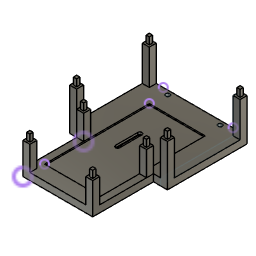
WRO BOTTOM LAYER_ (Autodesk Fusion 360 design; units mm, degrees)
Autodesk Fusion 360 part; units mm, degrees
note: some values were not read from the file. Set by a fixed rule: which sketch regions a step uses.
sketch "Sketch1" plane through (0, 0, 0) normal (1, 0, 0) x (0, 1, 0)
  line L0 (0, 0) -> (-25, 0)
  line L1 (-25, 0) -> (29, 0)
  line L2 (29, 0) -> (32, 0)
  line L3 (32, 0) -> (32, 30)
  line L4 (32, 30) -> (67, 30)
  line L5 (67, 30) -> (67, 35)
  line L6 (67, 35) -> (27, 35)
  line L7 (27, 35) -> (27, 5)
  line L8 (27, 5) -> (-25, 5)
  line L9 (-25, 5) -> (-25, 0)
  dimension "d1" = 25
  dimension "d2" = 54
  dimension "d3" = 3
  dimension "d4" = 30
  dimension "d5" = 35
  dimension "d6" = 5
  dimension "d7" = 40
  dimension "d8" = 30
  dimension "d9" = 52
  constraint coincident L0.start origin
  constraint horizontal L0
  constraint parallel L0 L1
  constraint parallel L1 L2
  constraint perpendicular L2 L3
  constraint perpendicular L3 L4
  constraint perpendicular L4 L5
  constraint perpendicular L5 L6
  constraint perpendicular L1 L7
  constraint perpendicular L7 L8
  measures "d1" distance of L0.start L0.end
  measures "d2" distance of L0.end L1.end
  measures "d3" distance of L1.end L2.end
  measures "d4" distance of L2.end L3.end
  measures "d5" distance of L3.end L4.end
  measures "d6" distance of L4.end L5.end
  measures "d7" distance of L5.end L6.end
  measures "d8" distance of L6.end L7.end
  measures "d9" distance of L7.end L8.end
extrude "Extrude1" add sketch "Sketch1" along normal blind 30 and the other way blind 30 makes body 1
sketch "Sketch2" plane through (0, 27, 0) normal (0, -1, 0) x (1, 0, 0)
  line L0 (-30, 5) -> (30, 5)
  line L1 (30, 5) -> (30, 35)
  line L2 (30, 35) -> (-30, 35)
  line L3 (-30, 35) -> (-30, 5)
  line L4 (-25, 5) -> (25, 5)
  line L5 (25, 5) -> (25, 30)
  line L6 (25, 30) -> (-25, 30)
  line L7 (-25, 30) -> (-25, 5)
  constraint horizontal L4
  constraint vertical L5
  constraint horizontal L6
  constraint vertical L7
  constraint coincident L0 L4.start
extrude "Extrude2" cut sketch "Sketch2" against normal blind 430 contours L0 L4 L5 L6 L7 bodies 1
sketch "Sketch3" plane through (0, 0, 5) normal (0, 0, 1) x (-1, 0, 0)
  line L0 (30, 25) -> (-30, 25)
  line L1 (-30, 25) -> (-30, -27)
  line L2 (-30, -27) -> (-25, -27)
  line L3 (-25, -27) -> (-25, -32)
  line L4 (-25, -32) -> (25, -32)
  line L5 (25, -32) -> (25, -27)
  line L6 (25, -27) -> (30, -27)
  line L7 (30, -27) -> (30, 25)
  line L8 (30, 0) -> (20, 0)
  line L9 (20, 0) -> (20, -20)
  line L10 (20, -20) -> (-20, -20)
  line L11 (-20, -20) -> (-20, 55)
  line L12 (-20, 55) -> (20, 55)
  line L13 (20, 55) -> (20, -20)
  dimension "d16" = 10
  dimension "d17" = 40
  dimension "d18" = 75
  constraint coincident L7 L8.start
  constraint perpendicular L7 L8
  constraint perpendicular L8 L9
  constraint horizontal L10
  constraint vertical L11
  constraint horizontal L12
  constraint vertical L13
  measures "d16" distance of L8.start L8.end
  measures "d17" distance of L9.end L10.end
  measures "d18" distance of L9.end L12.end
sketch "Sketch4" plane through (0, -25, 0) normal (0, -1, 0) x (1, 0, 0)
  line L0 (-30, 0) -> (30, 0)
  line L1 (30, 0) -> (30, 5)
  line L2 (30, 5) -> (-30, 5)
  line L3 (-30, 5) -> (-30, 0)
  line L4 (-30, 0) -> (-25, 0)
  line L5 (-25, 0) -> (25, 0)
  line L6 (25, 0) -> (25, 5)
  line L7 (25, 5) -> (-25, 5)
  line L8 (-25, 5) -> (-25, 0)
  dimension "d19" = 5
  dimension "d20" = 50
  dimension "d21" = 5
  constraint coincident L0.start L3.end
  constraint perpendicular L3 L4
  constraint horizontal L5
  constraint vertical L6
  constraint horizontal L7
  constraint vertical L8
  measures "d19" distance of L0.start L4.end
  measures "d20" distance of L4.end L5.end
  measures "d21" distance of L4.end L7.end
extrude "Extrude3" add sketch "Sketch4" along normal blind 43.5 contours L0 L2 L5 L6 L7 L8 bodies 1
extrude "Extrude4" cut sketch "Sketch3" against normal blind 1 contours L0 L9 L10 L11 L13 | L0 L11 L12 L13 bodies 1
sketch "Sketch5" plane through (30, 0, 0) normal (1, 0, 0) x (0, 1, 0)
  line L0 (-25, 5) -> (-25, 0)
  line L1 (-25, 0) -> (32, 0)
  line L2 (32, 0) -> (32, 30)
  line L3 (32, 30) -> (67, 30)
  line L4 (67, 30) -> (67, 35)
  line L5 (67, 35) -> (27, 35)
  line L6 (27, 35) -> (27, 5)
  line L7 (27, 5) -> (-25, 5)
  line L8 (67, 30) -> (62, 30)
  line L9 (62, 30) -> (62, 5)
  line L10 (62, 5) -> (67, 5)
  line L11 (67, 5) -> (67, 30)
  line L12 (62, 5) -> (78, 5)
  line L13 (78, 5) -> (78, 10)
  line L14 (78, 10) -> (62, 10)
  line L15 (62, 10) -> (62, 5)
  dimension "d26" = 5
  dimension "d27" = 25
  dimension "d28" = 16
  dimension "d29" = 5
  constraint horizontal L8
  constraint vertical L9
  constraint horizontal L10
  constraint vertical L11
  constraint coincident L3.end L4.start
  constraint horizontal L12
  constraint vertical L13
  constraint horizontal L14
  constraint vertical L15
  measures "d26" distance of L3.end L8.end
  measures "d27" distance of L3.end L10.end
  measures "d28" distance of L9.end L12.end
  measures "d29" distance of L9.end L14.end
extrude "Extrude5" add sketch "Sketch5" against normal blind 60 contours L3 L8 L9 L11 L14 | L9 L10 L11 L12 L14 L15 | L11 L12 L13 L14 bodies 1
sketch "Sketch6" plane through (30, 0, 0) normal (1, 0, 0) x (0, 1, 0)
  line L0 (-25, 5) -> (-25, 0)
  line L1 (-25, 0) -> (32, 0)
  line L2 (32, 0) -> (32, 30)
  line L3 (32, 30) -> (62, 30)
  line L4 (62, 30) -> (62, 5)
  line L5 (62, 5) -> (78, 5)
  line L6 (78, 5) -> (78, 10)
  line L7 (78, 10) -> (67, 10)
  line L8 (67, 10) -> (67, 35)
  line L9 (67, 35) -> (27, 35)
  line L10 (27, 35) -> (27, 5)
  line L11 (27, 5) -> (-25, 5)
  line L12 (62, 30) -> (99.4682, 30)
  line L13 (99.4682, 30) -> (99.4682, 1.0455)
  line L14 (99.4682, 1.0455) -> (62, 1.0455)
  line L15 (62, 1.0455) -> (62, 30)
  constraint horizontal L12
  constraint vertical L13
  constraint horizontal L14
  constraint vertical L15
  constraint coincident L3.end L4.start
extrude "Extrude6" cut sketch "Sketch6" against normal blind 5 contours L4 L5 L6 L7 L8 L12 L15 bodies 1
sketch "Sketch7" plane through (-30, 0, 0) normal (-1, 0, 0) x (0, -1, 0)
  line L0 (25, 0) -> (25, 5)
  line L1 (25, 5) -> (-27, 5)
  line L2 (-27, 5) -> (-27, 35)
  line L3 (-27, 35) -> (-67, 35)
  line L4 (-67, 35) -> (-67, 10)
  line L5 (-67, 10) -> (-78, 10)
  line L6 (-78, 10) -> (-78, 5)
  line L7 (-78, 5) -> (-62, 5)
  line L8 (-62, 5) -> (-62, 30)
  line L9 (-62, 30) -> (-32, 30)
  line L10 (-32, 30) -> (-32, 0)
  line L11 (-32, 0) -> (25, 0)
  line L12 (-62, 30) -> (-89.4119, 30)
  line L13 (-89.4119, 30) -> (-89.4119, -1.5433)
  line L14 (-89.4119, -1.5433) -> (-62, -1.5433)
  line L15 (-62, -1.5433) -> (-62, 30)
  constraint horizontal L12
  constraint vertical L13
  constraint horizontal L14
  constraint vertical L15
  constraint coincident L8.end L9.start
extrude "Extrude7" cut sketch "Sketch7" against normal blind 5 contours L4 L5 L6 L7 L8 L12 L15 bodies 1
sketch "Sketch8" plane through (0, 67, 0) normal (0, 1, 0) x (-1, 0, 0)
  line L0 (25, 30) -> (30, 30)
  line L1 (30, 30) -> (30, 35)
  line L2 (30, 35) -> (-30, 35)
  line L3 (-30, 35) -> (-30, 30)
  line L4 (-30, 30) -> (-25, 30)
  line L5 (-25, 30) -> (-25, 10)
  line L6 (-25, 10) -> (25, 10)
  line L7 (25, 10) -> (25, 30)
  line L8 (-25, 10) -> (-20, 10)
  line L9 (-20, 10) -> (20, 10)
  line L10 (20, 10) -> (20, 30)
  line L11 (20, 30) -> (-20, 30)
  line L12 (-20, 30) -> (-20, 10)
  dimension "d36" = 5
  dimension "d37" = 40
  constraint coincident L5.end L6.start
  constraint perpendicular L5 L8
  constraint horizontal L9
  constraint vertical L10
  constraint horizontal L11
  constraint vertical L12
  measures "d36" distance of L5.end L8.end
  measures "d37" distance of L8.end L9.end
extrude "Extrude8" cut sketch "Sketch8" against normal blind 16 contours L6 L9 L10 L11 L12 bodies 1
sketch "Sketch9" plane through (0, 0, 10) normal (0, 0, 1) x (-1, 0, 0)
  line L0 (25, -78) -> (25, -67)
  line L1 (25, -67) -> (20, -67)
  line L2 (20, -67) -> (20, -62)
  line L3 (20, -62) -> (-20, -62)
  line L4 (-20, -62) -> (-20, -67)
  line L5 (-20, -67) -> (-25, -67)
  line L6 (-25, -67) -> (-25, -78)
  line L7 (-25, -78) -> (25, -78)
  line L8 (-14, -62) -> (-14, -69.25)
  line L9 (-14, -69.25) -> (-14, -70)
  line L10 (-25, -70.7379) -> (0, -70.7379)
  line L11 (0, -70.7379) -> (-7.25, -70.7379)
  line L12 (-14, -70) -> (-7.25, -70)
  line L13 (-7.25, -70) -> (-7.25, -70.7379)
  circle A0 centre (-7.25, -70) radius 0.75
  line L14 (-7.25, -70) -> (7.25, -70)
  circle A1 centre (7.25, -70) radius 0.75
  dimension "d40" = 7.25
  dimension "d41" = 0.75
  dimension "d42" = 25
  dimension "d43" = 7.25
  dimension "d44" = 1.5
  dimension "d45" = 14.5
  dimension "d46" = 1.5
  constraint vertical L8
  constraint coincident L3 L8.start
  constraint perpendicular L7 L9
  constraint coincident L6 L10.start
  constraint perpendicular L0 L10
  constraint parallel L10 L11
  constraint perpendicular L9 L12
  constraint perpendicular L11 L13
  constraint coincident L12.end L13.start
  constraint perpendicular L13 L14
  constraint coincident L14.end A1.centre
  measures "d40" distance of L8.start L8.end
  measures "d41" distance of L8.end L9.end
  measures "d42" distance of L10.start L10.end
  measures "d43" distance of L10.end L11.end
  measures "d44" diameter of A0
  measures "d45" distance of L12.end L14.end
  measures "d46" diameter of A1
extrude "Extrude9" cut sketch "Sketch9" against normal blind 1000000 contours L10 L12 L13 A0 | L10 L11 L13 A0 L14 | L12 A0 L14 | A1 bodies 1
sketch "Sketch10" plane through (0, 0, 5) normal (0, 0, 1) x (-1, 0, 0)
  line L0 (-20, -20) -> (-20, 55)
  line L1 (-20, 55) -> (20, 55)
  line L2 (20, 55) -> (20, -20)
  line L3 (20, -20) -> (-20, -20)
  line L4 (-25, 25) -> (-30, 25)
  line L5 (-30, 25) -> (-30, -27)
  line L6 (-30, -27) -> (-25, -27)
  line L7 (-25, -27) -> (-25, -32)
  line L8 (-25, -32) -> (25, -32)
  line L9 (25, -32) -> (25, -27)
  line L10 (25, -27) -> (30, -27)
  line L11 (30, -27) -> (30, 25)
  line L12 (30, 25) -> (25, 25)
  line L13 (25, 25) -> (25, 68.5)
  line L14 (25, 68.5) -> (-25, 68.5)
  line L15 (-25, 68.5) -> (-25, 25)
  line L16 (15.6178, -32) -> (15.6178, -29)
  line L17 (15.6178, -29) -> (-84.3822, -29)
  line L18 (15.6178, -29) -> (37, -29)
  line L19 (25, -29) -> (0, -29)
  line L20 (0, -29) -> (18.75, -29)
  line L21 (18.75, -29) -> (-18.75, -29)
  circle A0 centre (18.75, -29) radius 1
  circle A1 centre (-18.75, -29) radius 1
  dimension "d49" = 3
  dimension "d50" = 100
  dimension "d51" = 25
  dimension "d52" = 18.75
  dimension "d53" = 37.5
  dimension "d54" = 2
  dimension "d55" = 2
  constraint coincident L8 L16.start
  constraint perpendicular L8 L16
  constraint perpendicular L16 L17
  constraint perpendicular L16 L18
  constraint coincident L18 L19.start
  constraint coincident L9 L19.start
  constraint perpendicular L7 L19
  constraint horizontal L20
  constraint perpendicular L16 L21
  constraint coincident L20.end L21.start
  constraint coincident L21.end A1.centre
  measures "d49" distance of L16.start L16.end
  measures "d50" distance of L16.end L17.end
  measures "d51" distance of L19.start L19.end
  measures "d52" distance of L19.end L20.end
  measures "d53" distance of L20.end L21.end
  measures "d54" diameter of A0
  measures "d55" diameter of A1
extrude "Extrude10" cut sketch "Sketch10" against normal blind 1000 contours L17 L21 A1 | L17 L21 A1 | L18 L19 L20 L21 A0 | L18 L19 L20 L21 A0 bodies 1
sketch "Sketch11" plane through (0, 0, 5) normal (0, 0, 1) x (-1, 0, 0)
  circle A0 centre (-18.75, -29) radius 1
  circle A1 centre (18.75, -29) radius 1
  line L0 (-20, -20) -> (-20, 55)
  line L1 (-20, 55) -> (20, 55)
  line L2 (20, 55) -> (20, -20)
  line L3 (20, -20) -> (-20, -20)
  line L4 (-25, 25) -> (-30, 25)
  line L5 (-30, 25) -> (-30, -27)
  line L6 (-30, -27) -> (-25, -27)
  line L7 (-25, -27) -> (-25, -32)
  line L8 (-25, -32) -> (25, -32)
  line L9 (25, -32) -> (25, -27)
  line L10 (25, -27) -> (30, -27)
  line L11 (30, -27) -> (30, 25)
  line L12 (30, 25) -> (25, 25)
  line L13 (25, 25) -> (25, 68.5)
  line L14 (25, 68.5) -> (-25, 68.5)
  line L15 (-25, 68.5) -> (-25, 25)
  circle A2 centre (18.75, -29) radius 1.5
  circle A3 centre (-18.75, -29) radius 1.5
  dimension "d58" = 3
  dimension "d59" = 3
  constraint concentric A1 A2
  constraint concentric A0 A3
  measures "d58" diameter of A2
  measures "d59" diameter of A3
extrude "Extrude11" cut sketch "Sketch11" against normal blind 2.5 contours A2 | A3 bodies 1
extrude "Extrude12" add 1 faces at (-6.6667, -5, 4) along direction (0, 0, 1) blind 1 on bodies 1 bodies 1
sketch "Sketch12" plane through (0, 0, 5) normal (0, 0, 1) x (-1, 0, 0)
  circle A0 centre (18.75, -29) radius 1.5
  circle A1 centre (-18.75, -29) radius 1.5
  line L0 (-25, 25) -> (-30, 25)
  line L1 (-30, 25) -> (-30, -27)
  line L2 (-30, -27) -> (-25, -27)
  line L3 (-25, -27) -> (-25, -32)
  line L4 (-25, -32) -> (25, -32)
  line L5 (25, -32) -> (25, -27)
  line L6 (25, -27) -> (30, -27)
  line L7 (30, -27) -> (30, 25)
  line L8 (30, 25) -> (25, 25)
  line L9 (25, 25) -> (25, 68.5)
  line L10 (25, 68.5) -> (-25, 68.5)
  line L11 (-25, 68.5) -> (-25, 25)
  line L12 (18.75, -29) -> (17.25, -29)
  line L13 (17.25, -29) -> (5.725, -29)
  line L14 (5.725, -29) -> (5.725, 21)
  circle A2 centre (5.7328, 20) radius 1
  circle A3 centre (5.7328, 20) radius 1
  line L15 (5.7328, 20) -> (4.7328, 20)
  line L16 (4.7328, 20) -> (6.7328, 20)
  line L17 (6.7328, 20) -> (6.7328, 4)
  line L18 (6.7328, 4) -> (4.7328, 4)
  line L19 (4.7328, 4) -> (4.7328, 20)
  circle A4 centre (5.7328, 4) radius 1
  dimension "d64" = 11.525
  dimension "d65" = 50
  dimension "d66" = 2
  dimension "d67" = 2
  dimension "d68" = 16
  dimension "d69" = 2
  constraint coincident A0.centre L12.start
  constraint coincident A0 L12.end
  constraint horizontal L12
  constraint parallel L12 L13
  constraint perpendicular L13 L14
  constraint coincident L14.end A2
  constraint concentric A2 A3
  constraint coincident A2.centre A3.centre
  constraint coincident A3 L15.end
  constraint perpendicular L14 L15
  constraint horizontal L16
  constraint vertical L17
  constraint horizontal L18
  constraint vertical L19
  constraint midpoint L18 A4.centre
  measures "d64" distance of L12.end L13.end
  measures "d65" distance of L13.end L14.end
  measures "d66" diameter of A2
  measures "d67" distance of L15.end L16.end
  measures "d68" distance of L15.end L18.end
  measures "d69" diameter of A4
extrude "Extrude13" cut sketch "Sketch12" against normal blind 10000 contours L14 L18 A4 | L14 L18 A4 | L14 L18 A4 | L14 L18 A4 | L14 A2 A3 L19 A4 | L14 A2 A3 L17 A4 | L14 A2 A3 L15 L16 | L14 A2 A3 L15 L16 | L14 A2 A3 L15 L16 | L14 A2 A3 L15 L16 bodies 1
sketch "Sketch13" plane through (0, 0, 5) normal (0, 0, 1) x (-1, 0, 0)
  line L0 (4.7328, 4) -> (4.7328, 20)
  arc A0 (6.7328, 20) -> (4.7328, 20) centre (5.7328, 20) ccw
  line L1 (6.7328, 20) -> (6.7328, 4)
  arc A1 (4.7328, 4) -> (6.7328, 4) centre (5.7328, 4) ccw
  circle A2 centre (18.75, -29) radius 1.5
  circle A3 centre (-18.75, -29) radius 1.5
  line L2 (-25, 25) -> (-30, 25)
  line L3 (-30, 25) -> (-30, -27)
  line L4 (-30, -27) -> (-25, -27)
  line L5 (-25, -27) -> (-25, -32)
  line L6 (-25, -32) -> (25, -32)
  line L7 (25, -32) -> (25, -27)
  line L8 (25, -27) -> (30, -27)
  line L9 (30, -27) -> (30, 25)
  line L10 (30, 25) -> (25, 25)
  line L11 (25, 25) -> (25, 68.5)
  line L12 (25, 68.5) -> (-25, 68.5)
  line L13 (-25, 68.5) -> (-25, 25)
  circle A4 centre (5.7328, 20) radius 1.5
  circle A5 centre (5.7328, 4) radius 1.5
  line L14 (5.7328, 4) -> (7.2328, 4)
  line L15 (7.2328, 4) -> (4.2328, 4)
  line L16 (4.2328, 4) -> (4.2328, 20)
  line L17 (4.2328, 20) -> (7.2328, 20)
  line L18 (7.2328, 20) -> (7.2328, 4)
  dimension "d72" = 3
  dimension "d73" = 3
  dimension "d74" = 3
  dimension "d75" = 16
  constraint concentric A0 A4
  constraint concentric A1 A5
  constraint coincident A1.centre A5.centre
  constraint coincident A5 L14.end
  constraint perpendicular L1 L14
  constraint horizontal L15
  constraint vertical L16
  constraint horizontal L17
  constraint vertical L18
  measures "d72" diameter of A4
  measures "d73" diameter of A5
  measures "d74" distance of L14.end L15.end
  measures "d75" distance of L14.end L17.end
extrude "Extrude14" cut sketch "Sketch13" against normal blind 2.5 contours L0 A5 L15 | A1 A5 L14 L15 | L0 A4 A5 L16 | L1 A5 L14 L15 | L0 A4 L17 | L1 A4 A5 L18 | A0 A4 L17 | L1 A4 L17 bodies 1
sketch "Sketch14" plane through (0, 0, 5) normal (0, 0, 1) x (-1, 0, 0)
  line L0 (7.2328, 20) -> (7.2328, 4)
  arc A0 (4.2328, 4) -> (7.2328, 4) centre (5.7328, 4) ccw
  line L1 (4.2328, 4) -> (4.2328, 20)
  arc A1 (7.2328, 20) -> (4.2328, 20) centre (5.7328, 20) ccw
  circle A2 centre (18.75, -29) radius 1.5
  circle A3 centre (-18.75, -29) radius 1.5
  line L2 (-25, 25) -> (-30, 25)
  line L3 (-30, 25) -> (-30, -27)
  line L4 (-30, -27) -> (-25, -27)
  line L5 (-25, -27) -> (-25, -32)
  line L6 (-25, -32) -> (25, -32)
  line L7 (25, -32) -> (25, -27)
  line L8 (25, -27) -> (30, -27)
  line L9 (30, -27) -> (30, 25)
  line L10 (30, 25) -> (25, 25)
  line L11 (25, 25) -> (25, 68.5)
  line L12 (25, 68.5) -> (-25, 68.5)
  line L13 (-25, 68.5) -> (-25, 25)
  line L14 (30, -20) -> (20, -20)
  line L15 (20, -20) -> (20, -32)
  line L16 (20, -32) -> (20, -12)
  line L17 (20, -12) -> (-20, -12)
  line L18 (-20, -12) -> (-20, 63)
  line L19 (-20, 63) -> (20, 63)
  line L20 (20, 63) -> (20, -12)
  dimension "d78" = 10
  dimension "d79" = 20
  dimension "d80" = 40
  dimension "d81" = 75
  constraint coincident L9 L14.start
  constraint perpendicular L9 L14
  constraint coincident L6 L15.end
  constraint perpendicular L6 L15
  constraint perpendicular L6 L16
  constraint horizontal L17
  constraint vertical L18
  constraint horizontal L19
  constraint vertical L20
  measures "d78" distance of L14.start L14.end
  measures "d79" distance of L15.end L16.end
  measures "d80" distance of L16.end L17.end
  measures "d81" distance of L16.end L19.end
extrude "Extrude15" cut sketch "Sketch14" against normal blind 1 contours L17 L18 L19 L20 bodies 1
extrude "Extrude16" add 1 faces at (6.6667, -63, 4.3333) along direction (0, 1, 0) blind 5 on bodies 1 bodies 1
extrude "Extrude17" cut 1 faces at (-6.6667, 12, 4.3333) along direction (0, 1, 0) blind 5 on bodies 1 bodies 1
sketch "Sketch15" plane through (0, 27, 0) normal (0, -1, 0) x (1, 0, 0)
  line L0 (-25, 5) -> (-25, 30)
  line L1 (-25, 30) -> (25, 30)
  line L2 (25, 30) -> (25, 5)
  line L3 (25, 5) -> (30, 5)
  line L4 (30, 5) -> (30, 35)
  line L5 (30, 35) -> (-30, 35)
  line L6 (-30, 35) -> (-30, 5)
  line L7 (-30, 5) -> (-25, 5)
  line L8 (30, 30) -> (-30, 30)
  line L9 (-30, 30) -> (-30, 35)
  line L10 (-30, 35) -> (30, 35)
  line L11 (30, 35) -> (30, 30)
  constraint horizontal L8
  constraint vertical L9
  constraint horizontal L10
  constraint vertical L11
  constraint coincident L5.end L6.start
  constraint coincident L4 L8.start
extrude "Extrude18" add sketch "Sketch15" along normal blind 60 contours L1 L4 L5 L6 L8 L9 L10 L11 bodies 1
extrude "Extrude19" cut 1 faces at (-10, -33, 33.3333) along direction (0, 1, 0) blind 10 on bodies 1 bodies 1
sketch "Sketch16" plane through (30, 0, 0) normal (1, 0, 0) x (0, 1, 0)
  line L0 (-23, 35) -> (-23, 30)
  line L1 (-23, 30) -> (27, 30)
  line L2 (27, 30) -> (27, 5)
  line L3 (27, 5) -> (-25, 5)
  line L4 (-25, 5) -> (-25, 0)
  line L5 (-25, 0) -> (32, 0)
  line L6 (32, 0) -> (32, 30)
  line L7 (32, 30) -> (67, 30)
  line L8 (67, 30) -> (67, 35)
  line L9 (67, 35) -> (-23, 35)
  line L10 (-23, 30) -> (95.9668, 30)
  line L11 (95.9668, 30) -> (95.9668, 42.0724)
  line L12 (95.9668, 42.0724) -> (-23, 42.0724)
  line L13 (-23, 42.0724) -> (-23, 30)
  line L14 (94.8078, 30) -> (50.5333, 30)
  line L15 (50.5333, 30) -> (50.5333, -4.5202)
  line L16 (50.5333, -4.5202) -> (94.8078, -4.5202)
  line L17 (94.8078, -4.5202) -> (94.8078, 30)
  constraint horizontal L10
  constraint vertical L11
  constraint horizontal L12
  constraint vertical L13
  constraint coincident L0.end L1.start
  constraint horizontal L14
  constraint vertical L15
  constraint horizontal L16
  constraint vertical L17
  constraint coincident L10 L14.start
extrude "Extrude20" cut sketch "Sketch16" against normal blind 100 contours L0 L1 L7 L8 L9 L10 L13 L14 | L7 L10 L14 L15 L16 L17 bodies 1
sketch "Sketch17" plane through (0, 0, 30) normal (0, 0, 1) x (-1, 0, 0)
  line L0 (-25, -27) -> (-30, -27)
  line L1 (-30, -27) -> (-30, -32)
  line L2 (-30, -32) -> (-25, -32)
  line L3 (-25, -32) -> (-25, -27)
  line L4 (-30, -32) -> (-30, -30.75)
  line L5 (-30, -30.75) -> (-28.75, -30.75)
  line L6 (-28.75, -30.75) -> (-26.25, -30.75)
  line L7 (-26.25, -30.75) -> (-26.25, -28.25)
  line L8 (-26.25, -28.25) -> (-28.75, -28.25)
  line L9 (-28.75, -28.25) -> (-28.75, -30.75)
  line L10 (30, -32) -> (30, -30.75)
  line L11 (30, -30.75) -> (28.75, -30.75)
  line L12 (28.75, -30.75) -> (26.25, -30.75)
  line L13 (26.25, -30.75) -> (26.25, -28.25)
  line L14 (26.25, -28.25) -> (28.75, -28.25)
  line L15 (28.75, -28.25) -> (28.75, -30.75)
  dimension "d94" = 1.25
  dimension "d95" = 1.25
  dimension "d96" = 2.5
  dimension "d97" = 2.5
  dimension "d98" = 1.25
  dimension "d99" = 1.25
  dimension "d100" = 2.5
  dimension "d101" = 2.5
  constraint coincident L1.end L2.start
  constraint perpendicular L2 L4
  constraint perpendicular L4 L5
  constraint horizontal L6
  constraint vertical L7
  constraint horizontal L8
  constraint vertical L9
  constraint vertical L10
  constraint perpendicular L10 L11
  constraint horizontal L12
  constraint vertical L13
  constraint horizontal L14
  constraint vertical L15
  measures "d94" distance of L1.end L4.end
  measures "d95" distance of L4.end L5.end
  measures "d96" distance of L5.end L6.end
  measures "d97" distance of L5.end L8.end
  measures "d98" distance of L10.start L10.end
  measures "d99" distance of L10.end L11.end
  measures "d100" distance of L11.end L12.end
  measures "d101" distance of L11.end L14.end
extrude "Extrude21" add sketch "Sketch17" along normal blind 5 contours L6 L7 L8 L9 | L12 L13 L14 L15 bodies 1
sketch "Sketch18" plane through (0, 0, 5) normal (0, 0, 1) x (-1, 0, 0)
  line L0 (-20, -17) -> (-20, 58)
  line L1 (-20, 58) -> (20, 58)
  line L2 (20, 58) -> (20, -17)
  line L3 (20, -17) -> (-20, -17)
  circle A0 centre (18.75, -29) radius 1.5
  circle A1 centre (-18.75, -29) radius 1.5
  line L4 (-25, 25) -> (-30, 25)
  line L5 (-30, 25) -> (-30, -27)
  line L6 (-30, -27) -> (-25, -27)
  line L7 (-25, -27) -> (-25, -32)
  line L8 (-25, -32) -> (25, -32)
  line L9 (25, -32) -> (25, -27)
  line L10 (25, -27) -> (30, -27)
  line L11 (30, -27) -> (30, 25)
  line L12 (30, 25) -> (25, 25)
  line L13 (25, 25) -> (25, 68.5)
  line L14 (25, 68.5) -> (-25, 68.5)
  line L15 (-25, 68.5) -> (-25, 25)
  line L16 (-25, 68.5) -> (-20, 68.5)
  line L17 (-20, 68.5) -> (-20, 63.5)
  line L18 (-20, 63.5) -> (-25, 63.5)
  line L19 (-25, 63.5) -> (-25, 68.5)
  line L20 (25, 68.5) -> (20, 68.5)
  line L21 (20, 68.5) -> (20, 63.5)
  line L22 (20, 63.5) -> (25, 63.5)
  line L23 (25, 63.5) -> (25, 68.5)
  dimension "d104" = 5
  dimension "d105" = 5
  dimension "d106" = 5
  constraint horizontal L16
  constraint vertical L17
  constraint horizontal L18
  constraint vertical L19
  constraint coincident L14.end L15.start
  constraint horizontal L20
  constraint vertical L21
  constraint horizontal L22
  constraint vertical L23
  constraint coincident L13.end L14.start
  measures "d104" distance of L14.end L18.end
  measures "d105" distance of L13.end L20.end
  measures "d106" distance of L13.end L22.end
extrude "Extrude22" add sketch "Sketch18" along normal blind 17.5 contours L14 L15 L16 L17 L18 L19 | L13 L14 L20 L21 L22 L23 bodies 1
sketch "Sketch19" plane through (0, 0, 22.5) normal (0, 0, 1) x (-1, 0, 0)
  line L0 (25, 63.5) -> (25, 68.5)
  line L1 (25, 68.5) -> (20, 68.5)
  line L2 (20, 68.5) -> (20, 63.5)
  line L3 (20, 63.5) -> (25, 63.5)
  line L4 (25, 68.5) -> (25, 67.25)
  line L5 (25, 67.25) -> (23.75, 67.25)
  line L6 (23.75, 67.25) -> (21.25, 67.25)
  line L7 (21.25, 67.25) -> (21.25, 64.75)
  line L8 (21.25, 64.75) -> (23.75, 64.75)
  line L9 (23.75, 64.75) -> (23.75, 67.25)
  line L10 (-25, 68) -> (-25, 68.5)
  line L11 (-25, 68.5) -> (-25, 67.25)
  line L12 (-25, 67.25) -> (-23.75, 67.25)
  line L13 (-23.75, 67.25) -> (-21.25, 67.25)
  line L14 (-21.25, 67.25) -> (-21.25, 64.75)
  line L15 (-21.25, 64.75) -> (-23.75, 64.75)
  line L16 (-23.75, 64.75) -> (-23.75, 67.25)
  dimension "d109" = 1.25
  dimension "d110" = 1.25
  dimension "d111" = 2.5
  dimension "d112" = 2.5
  dimension "d113" = 0.5
  dimension "d114" = 1.25
  dimension "d115" = 1.25
  dimension "d116" = 2.5
  dimension "d117" = 2.5
  constraint coincident L0.end L1.start
  constraint coincident L0 L4.end
  constraint perpendicular L4 L5
  constraint horizontal L6
  constraint vertical L7
  constraint horizontal L8
  constraint vertical L9
  constraint vertical L10
  constraint parallel L10 L11
  constraint perpendicular L11 L12
  constraint horizontal L13
  constraint vertical L14
  constraint horizontal L15
  constraint vertical L16
  measures "d109" distance of L0.end L4.end
  measures "d110" distance of L4.end L5.end
  measures "d111" distance of L5.end L6.end
  measures "d112" distance of L5.end L8.end
  measures "d113" distance of L10.start L10.end
  measures "d114" distance of L10.end L11.end
  measures "d115" distance of L11.end L12.end
  measures "d116" distance of L12.end L13.end
  measures "d117" distance of L12.end L15.end
extrude "Extrude23" add sketch "Sketch19" along normal blind 5 contours L6 L7 L8 L9 | L13 L14 L15 L16 bodies 1
sketch "Sketch20" plane through (0, 0, 27.5) normal (0, 0, 1) x (-1, 0, 0)
  line L0 (23.75, 64.75) -> (23.75, 67.25)
  line L1 (23.75, 67.25) -> (21.25, 67.25)
  line L2 (21.25, 67.25) -> (21.25, 64.75)
  line L3 (21.25, 64.75) -> (23.75, 64.75)
  line L4 (23.75, 67.25) -> (21.25, 67.25)
  line L5 (21.25, 67.25) -> (21.25, 64.75)
  line L6 (21.25, 64.75) -> (23.75, 64.75)
  line L7 (23.75, 64.75) -> (23.75, 67.25)
  line L8 (23.75, 67.25) -> (23.65, 67.25)
  line L9 (23.65, 67.25) -> (23.65, 67.15)
  line L10 (23.65, 67.15) -> (21.35, 67.15)
  line L11 (21.35, 67.15) -> (21.35, 64.85)
  line L12 (21.35, 64.85) -> (23.65, 64.85)
  line L13 (23.65, 64.85) -> (23.65, 67.15)
  dimension "d120" = 0.1
  dimension "d121" = 0.1
  dimension "d122" = 2.3
  dimension "d123" = 2.3
  constraint horizontal L4
  constraint vertical L5
  constraint horizontal L6
  constraint vertical L7
  constraint coincident L2.end L3.start
  constraint coincident L0.end L1.start
  constraint horizontal L8
  constraint perpendicular L1 L9
  constraint horizontal L10
  constraint vertical L11
  constraint horizontal L12
  constraint vertical L13
  measures "d120" distance of L0.end L8.end
  measures "d121" distance of L8.end L9.end
  measures "d122" distance of L9.end L10.end
  measures "d123" distance of L9.end L12.end
extrude "Extrude24" cut sketch "Sketch20" against normal blind 5 bodies 1
sketch "Sketch21" plane through (0, 0, 27.5) normal (0, 0, 1) x (-1, 0, 0)
  line L0 (-23.75, 64.75) -> (-21.25, 64.75)
  line L1 (-21.25, 64.75) -> (-21.25, 67.25)
  line L2 (-21.25, 67.25) -> (-23.75, 67.25)
  line L3 (-23.75, 67.25) -> (-23.75, 64.75)
  line L4 (-21.25, 67.25) -> (-21.25, 67.15)
  line L5 (-21.25, 67.15) -> (-21.35, 67.15)
  line L6 (-21.35, 67.15) -> (-23.65, 67.15)
  line L7 (-23.65, 67.15) -> (-23.65, 64.85)
  line L8 (-23.65, 64.85) -> (-21.35, 64.85)
  line L9 (-21.35, 64.85) -> (-21.35, 67.15)
  dimension "d126" = 0.1
  dimension "d127" = 0.1
  dimension "d128" = 2.3
  dimension "d129" = 2.3
  constraint coincident L1.end L2.start
  constraint perpendicular L2 L4
  constraint perpendicular L4 L5
  constraint horizontal L6
  constraint vertical L7
  constraint horizontal L8
  constraint vertical L9
  measures "d126" distance of L1.end L4.end
  measures "d127" distance of L4.end L5.end
  measures "d128" distance of L5.end L6.end
  measures "d129" distance of L5.end L8.end
extrude "Extrude25" cut sketch "Sketch21" against normal blind 5 bodies 1
sketch "Sketch22" plane through (0, 0, 35) normal (0, 0, 1) x (-1, 0, 0)
  line L0 (28.75, -28.25) -> (26.25, -28.25)
  line L1 (26.25, -28.25) -> (26.25, -30.75)
  line L2 (26.25, -30.75) -> (28.75, -30.75)
  line L3 (28.75, -30.75) -> (28.75, -28.25)
  line L4 (28.75, -28.25) -> (28.75, -28.35)
  line L5 (28.75, -28.35) -> (28.65, -28.35)
  line L6 (28.65, -28.35) -> (26.35, -28.35)
  line L7 (26.35, -28.35) -> (26.35, -30.65)
  line L8 (26.35, -30.65) -> (28.65, -30.65)
  line L9 (28.65, -30.65) -> (28.65, -28.35)
  line L10 (-28.65, -28.35) -> (-26.35, -28.35)
  line L11 (-26.35, -28.35) -> (-26.35, -30.65)
  line L12 (-26.35, -30.65) -> (-28.65, -30.65)
  line L13 (-28.65, -30.65) -> (-28.65, -28.35)
  line L14 (-28.75, -28.25) -> (-26.25, -28.25)
  line L15 (-26.25, -28.25) -> (-26.25, -30.75)
  line L16 (-26.25, -30.75) -> (-28.75, -30.75)
  line L17 (-28.75, -30.75) -> (-28.75, -28.25)
  dimension "d132" = 0.1
  dimension "d133" = 0.1
  dimension "d134" = 2.3
  dimension "d135" = 2.3
  dimension "d138" = 2.3
  dimension "d139" = 2.3
  dimension "d140" = 2.5
  dimension "d141" = 2.5
  constraint coincident L0.start L3.end
  constraint perpendicular L0 L4
  constraint perpendicular L4 L5
  constraint horizontal L6
  constraint vertical L7
  constraint horizontal L8
  constraint vertical L9
  constraint horizontal L10
  constraint vertical L11
  constraint horizontal L12
  constraint vertical L13
  constraint horizontal L14
  constraint vertical L15
  constraint horizontal L16
  constraint vertical L17
  measures "d132" distance of L0.start L4.end
  measures "d133" distance of L4.end L5.end
  measures "d134" distance of L5.end L6.end
  measures "d135" distance of L5.end L8.end
  measures "d138" distance of L10.start L10.end
  measures "d139" distance of L10.start L12.end
  measures "d140" distance of L14.start L14.end
  measures "d141" distance of L14.start L16.end
extrude "Extrude26" cut sketch "Sketch22" against normal blind 5 bodies 1
sketch "Sketch23" plane through (30, 0, 0) normal (1, 0, 0) x (0, 1, 0)
  line L0 (32, 30) -> (27, 30)
  line L1 (27, 30) -> (27, 5)
  line L2 (27, 5) -> (-25, 5)
  line L3 (-25, 5) -> (-25, 0)
  line L4 (-25, 0) -> (32, 0)
  line L5 (32, 0) -> (32, 30)
sketch "Sketch24" plane through (0, 0, 5) normal (0, 0, 1) x (-1, 0, 0)
  circle A0 centre (-18.75, -29) radius 1.5
  circle A1 centre (18.75, -29) radius 1.5
  line L0 (-20, -17) -> (-20, 58)
  line L1 (-20, 58) -> (20, 58)
  line L2 (20, 58) -> (20, -17)
  line L3 (20, -17) -> (-20, -17)
  line L4 (-20, 68.5) -> (-20, 63.5)
  line L5 (-20, 63.5) -> (-25, 63.5)
  line L6 (-25, 63.5) -> (-25, 25)
  line L7 (-25, 25) -> (-30, 25)
  line L8 (-30, 25) -> (-30, -27)
  line L9 (-30, -27) -> (-25, -27)
  line L10 (-25, -27) -> (-25, -32)
  line L11 (-25, -32) -> (25, -32)
  line L12 (25, -32) -> (25, -27)
  line L13 (25, -27) -> (30, -27)
  line L14 (30, -27) -> (30, 25)
  line L15 (30, 25) -> (25, 25)
  line L16 (25, 25) -> (25, 63.5)
  line L17 (25, 63.5) -> (20, 63.5)
  line L18 (20, 63.5) -> (20, 68.5)
  line L19 (20, 68.5) -> (-20, 68.5)
  line L20 (-30, 25) -> (-25, 25)
  line L21 (-25, 25) -> (-25, 20)
  line L22 (-25, 20) -> (-30, 20)
  line L23 (-30, 20) -> (-30, 25)
  line L24 (30, 25) -> (25, 25)
  line L25 (25, 25) -> (25, 20)
  line L26 (25, 20) -> (30, 20)
  line L27 (30, 20) -> (30, 25)
  dimension "d146" = 5
  dimension "d147" = 5
  dimension "d148" = 5
  constraint horizontal L20
  constraint vertical L21
  constraint horizontal L22
  constraint vertical L23
  constraint coincident L7.end L8.start
  constraint horizontal L24
  constraint vertical L25
  constraint horizontal L26
  constraint vertical L27
  constraint coincident L14.end L15.start
  measures "d146" distance of L7.end L22.end
  measures "d147" distance of L14.end L15.end
  measures "d148" distance of L14.end L26.end
extrude "Extrude27" add sketch "Sketch24" along normal blind 26 contours L7 L8 L20 L21 L22 L23 | L14 L15 L24 L25 L26 L27 bodies 1
sketch "Sketch25" plane through (30, 0, 0) normal (1, 0, 0) x (0, 1, 0)
  line L0 (32, 30) -> (-25, 30)
  line L1 (-25, 30) -> (-20, 30)
  line L2 (-20, 30) -> (-20, 31)
  line L3 (-20, 31) -> (-25, 31)
  line L4 (-25, 31) -> (-25, 30)
  constraint horizontal L0
  constraint horizontal L1
  constraint vertical L2
  constraint horizontal L3
  constraint vertical L4
extrude "Extrude28" cut sketch "Sketch25" against normal blind 10000 bodies 1
sketch "Sketch26" plane through (0, 0, 30) normal (0, 0, 1) x (-1, 0, 0)
  line L0 (25, 25) -> (25, 20)
  line L1 (25, 20) -> (30, 20)
  line L2 (30, 20) -> (30, 25)
  line L3 (30, 25) -> (25, 25)
  line L4 (30, 20) -> (30, 21.35)
  line L5 (30, 21.35) -> (28.65, 21.35)
  line L6 (28.65, 21.35) -> (26.35, 21.35)
  line L7 (26.35, 21.35) -> (26.35, 23.65)
  line L8 (26.35, 23.65) -> (28.65, 23.65)
  line L9 (28.65, 23.65) -> (28.65, 21.35)
  line L10 (-30, 20) -> (-30, 21.325)
  line L11 (-30, 21.325) -> (-28.675, 21.325)
  line L12 (-28.675, 21.325) -> (-26.375, 21.325)
  line L13 (-26.375, 21.325) -> (-26.375, 23.625)
  line L14 (-26.375, 23.625) -> (-28.675, 23.625)
  line L15 (-28.675, 23.625) -> (-28.675, 21.325)
  dimension "d153" = 1.35
  dimension "d154" = 1.35
  dimension "d155" = 2.3
  dimension "d156" = 2.3
  dimension "d157" = 1.325
  dimension "d158" = 1.325
  dimension "d159" = 2.3
  dimension "d160" = 2.3
  constraint coincident L1.end L2.start
  constraint perpendicular L1 L4
  constraint perpendicular L4 L5
  constraint horizontal L6
  constraint vertical L7
  constraint horizontal L8
  constraint vertical L9
  constraint vertical L10
  constraint perpendicular L10 L11
  constraint horizontal L12
  constraint vertical L13
  constraint horizontal L14
  constraint vertical L15
  measures "d153" distance of L1.end L4.end
  measures "d154" distance of L4.end L5.end
  measures "d155" distance of L5.end L6.end
  measures "d156" distance of L5.end L8.end
  measures "d157" distance of L10.start L10.end
  measures "d158" distance of L10.end L11.end
  measures "d159" distance of L11.end L12.end
  measures "d160" distance of L11.end L14.end
extrude "Extrude29" add sketch "Sketch26" along normal blind 5 contours L6 L7 L8 L9 | L12 L13 L14 L15 bodies 1
sketch "Sketch27" plane through (0, 0, 5) normal (0, 0, 1) x (-1, 0, 0)
  line L0 (-20, -17) -> (-20, 58)
  line L1 (-20, 58) -> (20, 58)
  line L2 (20, -17) -> (-20, -17)
  circle A0 centre (18.75, -29) radius 1.5
  circle A1 centre (-18.75, -29) radius 1.5
  line L3 (-25, 25) -> (-25, 20)
  line L4 (-25, 20) -> (-30, 20)
  line L5 (-30, 20) -> (-30, -27)
  line L6 (-30, -27) -> (-25, -27)
  line L7 (-25, -27) -> (-25, -32)
  line L8 (25, -32) -> (25, -27)
  line L9 (25, -27) -> (30, -27)
  line L10 (30, -27) -> (30, 20)
  line L11 (30, 20) -> (25, 20)
  line L12 (25, 20) -> (25, 25)
  line L13 (25, 25) -> (25, 63.5)
  line L14 (25, 63.5) -> (20, 63.5)
  line L15 (20, 63.5) -> (20, 68.5)
  line L16 (20, 68.5) -> (-20, 68.5)
  line L17 (-20, 68.5) -> (-20, 63.5)
  line L18 (-20, 63.5) -> (-25, 63.5)
  line L19 (-25, 63.5) -> (-25, 25)
sketch "Sketch28" plane through (-25, 0, 0) normal (-1, 0, 0) x (0, -1, 0)
  line L0 (25, 5) -> (25, 0)
  line L1 (68.5, 0) -> (68.5, 22.5)
  line L2 (68.5, 22.5) -> (63.5, 22.5)
  line L3 (63.5, 22.5) -> (63.5, 5)
  line L4 (63.5, 5) -> (25, 5)
sketch "Sketch29" plane through (0, 0, 5) normal (0, 0, 1) x (-1, 0, 0)
  line L0 (25, 25) -> (20, 25)
  line L1 (20, 25) -> (20, 30)
  line L2 (20, 30) -> (25, 30)
  line L3 (25, 30) -> (25, 25)
  line L4 (-25, 25) -> (-20, 25)
  line L5 (-20, 25) -> (-20, 30)
  line L6 (-20, 30) -> (-25, 30)
  line L7 (-25, 30) -> (-25, 25)
  dimension "d164" = 5
  dimension "d165" = 5
  dimension "d166" = 5
  dimension "d167" = 5
  constraint horizontal L0
  constraint vertical L1
  constraint horizontal L2
  constraint vertical L3
  constraint horizontal L4
  constraint vertical L5
  constraint horizontal L6
  constraint vertical L7
  measures "d164" distance of L0.start L0.end
  measures "d165" distance of L0.start L2.end
  measures "d166" distance of L4.start L4.end
  measures "d167" distance of L4.start L6.end
extrude "Extrude30" add sketch "Sketch29" along normal blind 17.5 separate body makes body 2 at (25, -28.3333, 10.8333) makes body 3 at (-23.3333, -25, 10.8333)
sketch "Sketch30" plane through (0, 0, 22.5) normal (0, 0, 1) x (-1, 0, 0)
  line L0 (-25, 30) -> (-25, 25)
  line L1 (-25, 25) -> (-20, 25)
  line L2 (-20, 25) -> (-20, 30)
  line L3 (-20, 30) -> (-25, 30)
  line L4 (25, 30) -> (25, 28.675)
  line L5 (25, 28.675) -> (23.675, 28.675)
  line L6 (23.675, 28.675) -> (21.375, 28.675)
  line L7 (21.375, 28.675) -> (21.375, 26.375)
  line L8 (21.375, 26.375) -> (23.675, 26.375)
  line L9 (23.675, 26.375) -> (23.675, 28.675)
  line L10 (-25, 30) -> (-25, 28.675)
  line L11 (-25, 28.675) -> (-23.75, 28.675)
  line L12 (-23.75, 28.675) -> (-23.65, 28.675)
  line L13 (-23.65, 28.675) -> (-21.35, 28.675)
  line L14 (-21.35, 28.675) -> (-21.35, 26.375)
  line L15 (-21.35, 26.375) -> (-23.65, 26.375)
  line L16 (-23.65, 26.375) -> (-23.65, 28.675)
  dimension "d170" = 1.325
  dimension "d171" = 1.325
  dimension "d172" = 2.3
  dimension "d173" = 2.3
  dimension "d174" = 1.325
  dimension "d175" = 1.25
  dimension "d176" = 0.1
  dimension "d177" = 2.3
  dimension "d178" = 2.3
  constraint vertical L4
  constraint perpendicular L4 L5
  constraint horizontal L6
  constraint vertical L7
  constraint horizontal L8
  constraint vertical L9
  constraint coincident L0.start L3.end
  constraint perpendicular L3 L10
  constraint perpendicular L10 L11
  constraint horizontal L12
  constraint horizontal L13
  constraint vertical L14
  constraint horizontal L15
  constraint vertical L16
  measures "d170" distance of L4.start L4.end
  measures "d171" distance of L4.end L5.end
  measures "d172" distance of L5.end L6.end
  measures "d173" distance of L5.end L8.end
  measures "d174" distance of L0.start L10.end
  measures "d175" distance of L10.end L11.end
  measures "d176" distance of L11.end L12.end
  measures "d177" distance of L12.end L13.end
  measures "d178" distance of L12.end L15.end
extrude "Extrude31" add sketch "Sketch30" along normal blind 5 contours L6 L7 L8 L9 | L13 L14 L15 L16 bodies 2 3
extrude "Extrude32" add 1 faces at (-30, -4.3333, 1.6667) along direction (-1, 0, 0) blind 5 on bodies 1 bodies 1
extrude "Extrude33" add 2 faces at (-28.65, 29.8833, 33.3333) (-28.65, -22.8833, 31.6667) along direction (-1, 0, 0) blind 5 on bodies 1 bodies 1
extrude "Extrude34" add 1 faces at (30, -4.3333, 1.6667) along direction (1, 0, 0) blind 5 on bodies 1 bodies 1
extrude "Extrude35" add 1 faces at (28.65, 29.8833, 33.3333) along direction (1, 0, 0) blind 5 on bodies 1 bodies 1
extrude "Extrude36" add 1 faces at (28.675, -22.8583, 31.6667) along direction (1, 0, 0) blind 5 on bodies 1 bodies 1
extrude "Extrude37" cut 1 faces at (25, -23.3333, 21.6667) along direction (1, 0, 0) blind 5 on bodies 1 bodies 1
extrude "Extrude38" cut 1 faces at (25, 28.6667, 13.3333) along direction (1, 0, 0) blind 5 on bodies 1 bodies 1
extrude "Extrude39" cut 1 faces at (26.35, 29.1167, 33.3333) along direction (1, 0, 0) blind 5 on bodies 1 bodies 1
extrude "Extrude40" cut 1 faces at (26.375, -22.0917, 31.6667) along direction (1, 0, 0) blind 5 on bodies 1 bodies 1
extrude "Extrude41" cut 2 faces at (-25, -23.3333, 21.6667) (-25, 28.6667, 21.6667) along direction (-1, 0, 0) blind 5 on bodies 1 bodies 1
extrude "Extrude42" cut 2 faces at (-26.35, 29.1167, 33.3333) (-26.35, -22.1167, 31.6667) along direction (-1, 0, 0) blind 5 on bodies 1 bodies 1
extrude "Extrude43" cut 1 faces at (-22.1417, -27.9083, 27.5) along direction (0, 0, -1) blind 5 on bodies 3 bodies 3
extrude "Extrude44" cut 1 faces at (22.8833, -27.9083, 27.5) along direction (0, 0, -1) blind 5 on bodies 2 bodies 2
extrude "Extrude45" cut 1 faces at (32.1417, -22.8583, 35) along direction (0, 0, -1) blind 5 on bodies 1 bodies 1
sketch "Sketch31" plane through (0, 0, 22.5) normal (0, 0, 1) x (-1, 0, 0)
  line L0 (-25, 30) -> (-25, 25)
  line L1 (-25, 25) -> (-20, 25)
  line L2 (-20, 25) -> (-20, 30)
  line L3 (-20, 30) -> (-25, 30)
  line L4 (-25, 30) -> (-23.65, 30)
  line L5 (-23.65, 30) -> (-23.65, 28.65)
  line L6 (-23.65, 28.65) -> (-21.35, 28.65)
  line L7 (-21.35, 28.65) -> (-21.35, 26.35)
  line L8 (-21.35, 26.35) -> (-23.65, 26.35)
  line L9 (-23.65, 26.35) -> (-23.65, 28.65)
  line L10 (25, 30) -> (23.65, 30)
  line L11 (23.65, 30) -> (23.65, 28.65)
  line L12 (23.65, 28.65) -> (21.35, 28.65)
  line L13 (21.35, 28.65) -> (21.35, 26.35)
  line L14 (21.35, 26.35) -> (23.65, 26.35)
  line L15 (23.65, 26.35) -> (23.65, 28.65)
  dimension "d209" = 1.35
  dimension "d210" = 1.35
  dimension "d211" = 2.3
  dimension "d212" = 2.3
  dimension "d213" = 1.35
  dimension "d214" = 1.35
  dimension "d215" = 2.3
  dimension "d216" = 2.3
  constraint coincident L0.start L3.end
  constraint coincident L3 L4.end
  constraint perpendicular L4 L5
  constraint horizontal L6
  constraint vertical L7
  constraint horizontal L8
  constraint vertical L9
  constraint horizontal L10
  constraint perpendicular L10 L11
  constraint horizontal L12
  constraint vertical L13
  constraint horizontal L14
  constraint vertical L15
  measures "d209" distance of L0.start L4.end
  measures "d210" distance of L4.end L5.end
  measures "d211" distance of L5.end L6.end
  measures "d212" distance of L5.end L8.end
  measures "d213" distance of L10.start L10.end
  measures "d214" distance of L10.end L11.end
  measures "d215" distance of L11.end L12.end
  measures "d216" distance of L11.end L14.end
extrude "Extrude46" add sketch "Sketch31" along normal blind 5 contours L6 L7 L8 L9 | L12 L13 L14 L15 bodies 2 3
sketch "Sketch32" plane through (0, 0, 30) normal (0, 0, 1) x (-1, 0, 0)
  line L0 (-30, 20) -> (-30, 25)
  line L1 (-30, 25) -> (-35, 25)
  line L2 (-35, 25) -> (-35, 20)
  line L3 (-35, 20) -> (-30, 20)
  line L4 (-35, 25) -> (-33.65, 25)
  line L5 (-33.65, 25) -> (-33.65, 23.65)
  line L6 (-33.65, 23.65) -> (-31.35, 23.65)
  line L7 (-31.35, 23.65) -> (-31.35, 21.35)
  line L8 (-31.35, 21.35) -> (-33.65, 21.35)
  line L9 (-33.65, 21.35) -> (-33.65, 23.65)
  dimension "d219" = 1.35
  dimension "d220" = 1.35
  dimension "d221" = 2.3
  dimension "d222" = 2.3
  constraint coincident L1.end L2.start
  constraint perpendicular L2 L4
  constraint perpendicular L1 L5
  constraint horizontal L6
  constraint vertical L7
  constraint horizontal L8
  constraint vertical L9
  measures "d219" distance of L1.end L4.end
  measures "d220" distance of L4.end L5.end
  measures "d221" distance of L5.end L6.end
  measures "d222" distance of L5.end L8.end
extrude "Extrude47" add sketch "Sketch32" along normal blind 5 contours L6 L7 L8 L9 bodies 1
